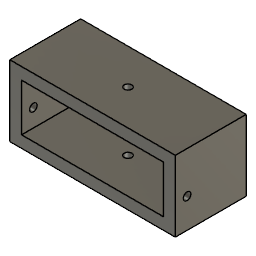
part - head1 (Autodesk Fusion 360 design; units mm, degrees)
Autodesk Fusion 360 part; units mm, degrees
sketch "Sketch1" plane through (0, 0, 0) normal (0, 1, 0) x (1, 0, 0)
  line L0 (35, -15) -> (-35, -15)
  line L1 (-35, -15) -> (-35, 15)
  line L2 (-35, 15) -> (35, 15)
  line L3 (35, 15) -> (35, -15)
  line L4 (35, -15) -> (-35, 15) construction
  line L5 (-35, -15) -> (35, 15) construction
  line L6 (-30, 10) -> (30, 10)
  line L7 (30, 10) -> (30, -10)
  line L8 (30, -10) -> (-30, -10)
  line L9 (-30, -10) -> (-30, 10)
  dimension "d1" = 70
  dimension "d2" = 30
  dimension "d3" = 5
  constraint horizontal L0
  constraint perpendicular L0 L1
  constraint parallel L0 L2
  constraint parallel L1 L3
  constraint coincident L4 origin
  constraint coincident L5 origin
  measures "d1" distance of L0.start L0.end
  measures "d2" distance of L0.end L1.end
extrude "Extrude1" add sketch "Sketch1" along normal mid plane 30
sketch "Sketch2" plane through (35, 0, 0) normal (1, 0, 0) x (0, 1, 0)
  line L0 (-15, -15) -> (15, -15)
  line L1 (15, -15) -> (15, 15)
  line L2 (15, 15) -> (-15, 15)
  line L3 (-15, 15) -> (-15, -15)
  circle A0 centre (-10, -2.5) radius 1.6
  dimension "d6" = 3.2
  dimension "d7" = 12.5
  dimension "d8" = 5
  measures "d6" diameter of A0
  measures "d7" distance of L0 A0.centre
  measures "d8" distance of L3 A0.centre
extrude "Extrude2" cut sketch "Sketch2" against normal blind 76 contours A0
sketch "Sketch3" plane through (0, 0, 15) normal (0, 0, 1) x (-1, 0, 0)
  line L0 (-35, 15) -> (-35, -15)
  line L1 (-35, -15) -> (35, -15)
  line L2 (35, -15) -> (35, 15)
  line L3 (35, 15) -> (-35, 15)
  circle A0 centre (0, 0) radius 1.6
  dimension "d11" = 3.2
  constraint coincident A0.centre origin
  measures "d11" diameter of A0
extrude "Extrude3" cut sketch "Sketch3" against normal blind 41 contours A0
equation "d7 = ( 25 / 2 ) * 1 mm"
